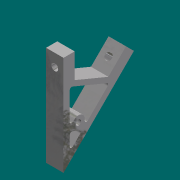
# Autodesk Inventor part: HBL45TS5hbl45ts5
Saved by Autodesk Inventor 2016 (Build 200138000, 138)
## iProperties
Category: PARTsolutions
Company: MISUMI
Created: 2016-02-10
Part Number: HBL45TS5hbl45ts5
Catalog Web Link: www.cadenas.de
Description: HBL45TS5, HBL45TD5, HBL135TS5, HBL135TD5-Brackets with Angle 45/135 Deg.
Vendor: MISUMI
Document SubType Name: Modeling
Designer: psAdmin
Manufacturer: MISUMI
Mass: 124.337 g
Surface Area: 80.2626 cm^2
Volume: 15.5422 cm^3
Density: 8 g/cm^3
Material: Stainless Steel
Appearance: Semi-Polished
PSOL_IDENT_0: {$CADENAS_DATA\23d-libs\misumi\metric\38_al_extrusions_blackets\5\hbl45ts5.prj},218 {VTYP=3D},{NB=HB
PSOL_IDENT_1: L45TS5hbl45ts5},{LINA=HBL45TS5hbl45ts5},{NN=HBL45TS5, HBL45TD5, HBL135TS5, HBL135TD5},{DATE=17.07.20
PSOL_IDENT_2: 15 10:47:02},{GEOMDATE=16.03.2009 12:27:00},{VERSION=},{LINEID=100},{LINESUBID=-1},{WBVAR=ALT1,ALT3}
PSOL_IDENT_3: {NB=HBL45TS5hbl45ts5},{LINA=HBL45TS5hbl45ts5},{KT=1},{PN=HBL45TS5},{TP=HBL45TS5},{MAT=JIS-A6N01SS-
PSOL_IDENT_4: T5},{ST=Anodizing},{TYPE=HBL45TS5},{FEAT=Brackets with Angle 45 Deg.},{SLOT=Slot Width 6 Frame},{ALT
PSOL_IDENT_5: 1=},{MASS=41},{AB=CBM5-14},{NOB=2},{AN=HNTT5-5},{NON=2},{AL=833},{W=14},{DIA=5.5},{ALT1OPT='','w/o C
PSOL_IDENT_6: (Mounting Holes for Cover)','-C','with C (Mounting Holes for Cover)'},{VER=5},{DIS=0.000},{VERS=1.0
PSOL_IDENT_7: 00},{ALT3=}
NN: HBL45TS5, HBL45TD5, HBL135TS5, HBL135TD5
NT: Brackets with Angle 45/135 Deg.
NB: HBL45TS5hbl45ts5
NBSYN: $PN.hbl45ts5
LINA: HBL45TS5hbl45ts5
PN: HBL45TS5
TP: HBL45TS5
MAT: A6N01SS-T5
ST: Anodizing
FEAT: Brackets with Angle 45 Deg.
SLOT: Slot Width 6 Frame
ALT1: w/o C (Mounting Holes for Cover)
MASS: 41
AB: CBM5-14
NOB: 2
AN: HNTT5-5
NON: 2
AL: 833
SUPPLIER: MISUMI
ARTICLENO: HBL45TS5hbl45ts5
BOMINFO: HBL45TS5hbl45ts5
CREATOR: CADENAS GmbH
Title: HBL45TS5hbl45ts5
Author: Cadenas PARTsolutions
Comments: Brackets with Angle 45/135 Deg.
Autodesk Inventor part; units mm, degrees
sketch "Sketch_1" plane through (0, 0, 0) normal (1, 0, 0) x (0, 1, 0)
  line L0 (0, 80) -> (0, 0)
  line L1 (0, 0) -> (56.5685, 56.5685)
  line L2 (56.5685, 56.5685) -> (50.2046, 62.9325)
  line L3 (50.2046, 62.9325) -> (36.0624, 48.7904)
  line L4 (36.0624, 48.7904) -> (9, 60)
  line L5 (9, 60) -> (9, 80)
  line L6 (9, 80) -> (0, 80)
  arc A0 (6.8931, 25.3806) -> (5, 23.933) centre (6.5, 23.933) ccw
  line L7 (5, 23.933) -> (5, 15.6924)
  arc A1 (5, 15.6924) -> (7.5607, 14.6317) centre (6.5, 15.6924) ccw
  line L8 (7.5607, 14.6317) -> (13.3877, 20.4587)
  arc A2 (13.3877, 20.4587) -> (13.0726, 22.821) centre (12.327, 21.5194) ccw
  arc A3 (13.0726, 22.821) -> (6.8931, 25.3806) centre (0, 0) ccw
  circle A4 centre (12, 28.9706) radius 2.1
  arc A5 (7.074, 56.4682) -> (5, 55.0824) centre (6.5, 55.0824) ccw
  line L9 (5, 55.0824) -> (5, 32.7559)
  arc A6 (5, 32.7559) -> (7.5929, 31.7285) centre (6.5, 32.7559) ccw
  line L10 (7.5929, 31.7285) -> (8.2843, 32.4639)
  arc A7 (17.0976, 28.8133) -> (8.2843, 32.4639) centre (12, 28.9706) ccw
  line L11 (17.0976, 28.8133) -> (17.0665, 27.8044)
  arc A8 (17.0665, 27.8044) -> (19.6264, 26.6975) centre (18.5657, 27.7581) ccw
  line L12 (19.6264, 26.6975) -> (35.4136, 42.4847)
  arc A9 (35.4136, 42.4847) -> (34.927, 44.9311) centre (34.3529, 43.5453) ccw
  line L13 (34.927, 44.9311) -> (7.074, 56.4682)
  constraints: 28 end point, 18 point on circle, 10 centre point
extrude "Extrusion1" add sketch "Sketch_1" along normal mid plane 14
sketch "Sketch2" plane through (-7, 50.2046, 62.9325) normal (0, -0.7071068, 0.7071068) x (1, 0, 0)
  point P0 (7, -10)
hole "Hole1" at (0, 43.1335, 55.8614) direction (0, 0.7071068, -0.7071068) diameter 5.5 depth 9
sketch "Sketch3" plane through (-7, 0, 80) normal (0, -1, 0) x (1, 0, 0)
  point P0 (7, -10)
hole "Hole2" at (0, 0, 70) direction (0, 1, 0) diameter 5.5 depth 9
ref_plane "bracket_to_dummy_XY" through (0, 0, 0) normal (0, 1, 0) x (1, 0, 0)
ref_plane "bracket_to_dummy_YZ" through (0, 0, 0) normal (1, 0, 0) x (0, 0, -1)
ref_plane "bracket_to_dummy_ZX" through (0, 0, 0) normal (0, 0, -1) x (0, 1, 0)
ref_plane "to_bolts_b_1_XY" through (0, 43.1335, 55.8614) normal (0, -0.7071068, 0.7071068) x (1, 0, 0)
ref_plane "to_bolts_b_1_YZ" through (0, 43.1335, 55.8614) normal (1, 0, 0) x (0, 0.7071068, 0.7071068)
ref_plane "to_bolts_b_1_ZX" through (0, 43.1335, 55.8614) normal (0, 0.7071068, 0.7071068) x (0, -0.7071068, 0.7071068)
ref_plane "to_bolts_base_b_1_XY" through (0, 9, 70) normal (0, 1, 0) x (1, 0, 0)
ref_plane "to_bolts_base_b_1_YZ" through (0, 9, 70) normal (1, 0, 0) x (0, 0, -1)
ref_plane "to_bolts_base_b_1_ZX" through (0, 9, 70) normal (0, 0, -1) x (0, 1, 0)
ref_plane "to_nuts_b_1_XY" through (0, 50.9117, 48.0833) normal (0, -0.7071068, 0.7071068) x (1, 0, 0)
ref_plane "to_nuts_b_1_YZ" through (0, 50.9117, 48.0833) normal (1, 0, 0) x (0, 0.7071068, 0.7071068)
ref_plane "to_nuts_b_1_ZX" through (0, 50.9117, 48.0833) normal (0, 0.7071068, 0.7071068) x (0, -0.7071068, 0.7071068)
ref_plane "to_nuts_base_b_1_XY" through (0, -2, 70) normal (0, 1, 0) x (1, 0, 0)
ref_plane "to_nuts_base_b_1_YZ" through (0, -2, 70) normal (1, 0, 0) x (0, 0, -1)
ref_plane "to_nuts_base_b_1_ZX" through (0, -2, 70) normal (0, 0, -1) x (0, 1, 0)
body "Solid1"
